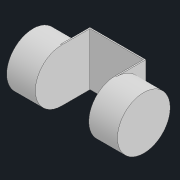
# Autodesk Inventor part: link1
Saved by Autodesk Inventor 2021 (Build 250183000, 183)
## iProperties
Created: 2021-07-10
Part Number: link1
Material: 一般
Document SubType Name: Modeling
Designer: yuta0
Density: 1 g/cm^3
Appearance: 既定
Author: yuta0
Autodesk Inventor part; units mm, degrees
ref_plane "YZ Plane" through (0, 0, 0) normal (1, 0, 0) x (0, 1, 0)
ref_plane "XZ Plane" through (0, 0, 0) normal (0, 1, 0) x (-1, 0, 0)
ref_plane "XY Plane" through (0, 0, 0) normal (0, 0, 1) x (1, 0, 0)
sketch "スケッチ1" plane through (0, 0, 0) normal (0, 0, 1) x (1, 0, 0)
  line L0 (71.7, -67.5) -> (-71.7, -67.5)
  line L1 (-71.7, -67.5) -> (-71.7, 67.5)
  line L2 (-71.7, 67.5) -> (71.7, 67.5)
  line L3 (71.7, 67.5) -> (71.7, -67.5)
  line L4 (71.7, -67.5) -> (-71.7, 67.5) construction
  line L5 (-71.7, -67.5) -> (71.7, 67.5) construction
  point P0 (0, 0)
  dimension "d0" = 135
  dimension "d1" = 143.4
  constraints: 12 end point, 2 midpoint, 2 parallel, 1 horizontal, 1 perpendicular
  measures "d0" distance of L0.end L1.end
  measures "d1" distance of L1.end L2.end
extrude "押し出し1" add sketch "スケッチ1" along normal blind 3
sketch "スケッチ2" plane through (0, 0, 3) normal (0, 0, 1) x (1, 0, 0)
  line L0 (-71.7, 67.5) -> (-71.7, -67.5) projected
  line L1 (71.7, 67.5) -> (-71.7, 67.5) projected
  line L2 (-71.7, -67.5) -> (-68.5, -67.5)
  line L3 (-68.5, -67.5) -> (-68.5, 67.5)
  line L4 (-68.5, 67.5) -> (-71.7, 67.5)
  line L5 (-71.7, 67.5) -> (-71.7, -67.5)
  line L6 (-71.7, -67.5) -> (71.7, -67.5) projected
  line L7 (71.7, -67.5) -> (68.5, -67.5)
  line L8 (68.5, -67.5) -> (68.5, 67.5)
  line L9 (68.5, 67.5) -> (71.7, 67.5)
  line L10 (71.7, 67.5) -> (71.7, -67.5)
  point P0 (0, 0)
  point P1 (71.7, 67.5)
  point P2 (68.5, -67.5)
  dimension "d4" = 3.2
  dimension "d5" = 3.2
  constraints: 16 end point, 4 parallel, 2 horizontal, 2 perpendicular, 2 point on line
  measures "d4" distance between parallel lines of L10 L8
  measures "d5" distance between parallel lines of L0 L3
extrude "押し出し2" add sketch "スケッチ2" along normal blind 140 contours L1 L3 L2 L0 | L1 L10 L6 L8
sketch "スケッチ3" plane through (71.7, -67.5, 0) normal (1, 0, 0) x (0, 0, -1)
  circle A0 centre (-75.5, 67.5) radius 67.5
  line L0 (-143, 0) -> (-143, 135) projected
  line L1 (0, 0) -> (-143, 0) projected
  line L2 (0, 135) -> (-143, 135) projected
  point P0 (0, 67.5)
  point P1 (-75.5, 0)
  point P2 (-143, 67.5)
  point P3 (-75.5, 135)
  constraints: 3 tangent, 1 centre point
extrude "押し出し3" cut sketch "スケッチ3" against normal through all contours A0 L0 L2 | L1 L0 A0
sketch "スケッチ4" plane through (71.7, -67.5, 0) normal (1, 0, 0) x (0, 0, -1)
  arc A0 (-75.5, 135) -> (-75.5, 0) centre (-75.5, 67.5) ccw projected
  circle A1 centre (-75.5, 67.5) radius 67.5
  point P0 (0, 67.5)
  point P1 (-75.5, 0)
  constraints: 1 coincident, 3 other
extrude "押し出し4" add sketch "スケッチ4" along normal blind 70
sketch "スケッチ5" plane through (-71.7, -67.5, 0) normal (-1, 0, 0) x (0, 0, 1)
  arc A0 (75.5, 0) -> (75.5, 135) centre (75.5, 67.5) ccw projected
  circle A1 centre (75.5, 67.5) radius 67.5
  point P0 (0, 67.5)
  constraints: 1 coincident, 3 other
extrude "押し出し5" add sketch "スケッチ5" along normal blind 70
move or copy body "移動1" bodies to move or copy 1 copy no translate (0, 0, -75.5)
